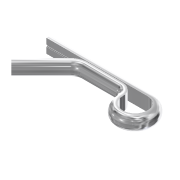
# Autodesk Inventor part: contra_pino_1
Saved by Autodesk Inventor 2012 SP2 (Build 160219200, 219)
## iProperties
Created: 2015-05-27
Part Number: contra_pino_1
Material: Default
Document SubType Name: Modeling
Designer: Projeto02
Density: 1 g/cm^3
Author: Projeto02
Autodesk Inventor part; units mm, degrees
ref_plane "YZ Plane" through (0, 0, 0) normal (1, 0, 0) x (0, 1, 0)
ref_plane "XZ Plane" through (0, 0, 0) normal (0, 1, 0) x (-1, 0, 0)
ref_plane "XY Plane" through (0, 0, 0) normal (0, 0, 1) x (1, 0, 0)
sketch "Esboço1" plane through (0, 0, 0) normal (0, 0, 1) x (1, 0, 0)
  line L0 (0, 0) -> (20.55, 0)
  line L1 (23, -2.45) -> (23, -2.55)
  line L2 (15.55, -0.1) -> (8.4497, -0.1)
  line L3 (5.9749, -1.1251) -> (0, -7.1)
  line L4 (18, -2.55) -> (18, -2.55)
  line L5 (20.45, -5) -> (20.55, -5)
  arc A0 (23, -2.45) -> (20.55, 0) centre (20.55, -2.45) ccw
  arc A1 (20.55, -5) -> (23, -2.55) centre (20.55, -2.55) ccw
  arc A2 (18, -2.55) -> (20.45, -5) centre (20.45, -2.55) ccw
  arc A3 (18, -2.55) -> (15.55, -0.1) centre (15.55, -2.55) ccw
  arc A4 (8.4497, -0.1) -> (5.9749, -1.1251) centre (8.4497, -3.6) ccw
  point P0 (23, 0)
  point P1 (18, -0.1)
  point P2 (7, -0.1)
  dimension "d0" = 23
  dimension "d1" = 135
  dimension "d2" = 5
  dimension "d3" = 5
  dimension "d4" = 11
  dimension "d5" = 0.1
  dimension "d6" = 2.45
  dimension "d10" = 3.5
  constraints: 12 end point, 10 point on circle, 10 tangent, 6 point on line, 5 centre point, 3 equal radius, 2 parallel, 1 horizontal, 1 vertical, 1 vertical alignment
  measures "d0" distance of L0.start point (23, 0)
  measures "d1" angle of L2 L3
  measures "d2" distance between parallel lines of L0 L5
  measures "d3" distance between parallel lines of L1 L4
  measures "d4" distance of point (18, -0.1) point (7, -0.1)
  measures "d5" distance between parallel lines of L0 L2
  measures "d6" radius of A0
  measures "d10" radius of A4
sketch "Esboço2" plane through (0, 0, 0) normal (1, 0, 0) x (0, 1, 0)
  line L0 (0, -1.5038) -> (0, 1.2962)
  line L1 (0, 1.2962) -> (0.15, 1.2962)
  line L2 (1.4, 0.0462) -> (1.4, -0.2538)
  line L3 (0.15, -1.5038) -> (0, -1.5038)
  arc A0 (1.4, 0.0462) -> (0.15, 1.2962) centre (0.15, 0.0462) ccw
  arc A1 (0.15, -1.5038) -> (1.4, -0.2538) centre (0.15, -0.2538) ccw
  dimension "d13" = 2.8
  dimension "d14" = 90
  dimension "d15" = 90
  dimension "d16" = 1.4
  dimension "d17" = 1.25
  constraints: 8 end point, 4 point on circle, 4 tangent, 2 centre point, 1 equal radius, 1 parallel
  measures "d13" distance of L0.start L0.end
  measures "d14" angle of L2 L3
  measures "d15" angle of L1 L2
  measures "d16" distance between parallel lines of L0 L2
  measures "d17" radius of A0
sweep "Varredura1" add profiles "Esboço2" path "Esboço1"
sketch "Esboço3" plane through (0, 0, -1.5038) normal (-1, 0, 0) x (0, 0, 1)
  line L0 (0, 0) -> (2.8, 0) projected
  circle A0 centre (1.4, -0.05) radius 0.2272
  point P0 (1.5038, 0)
  dimension "d18" = 1.4
  dimension "d19" = 2.8
  dimension "d20" = 0.05
  constraints: 1 centre point
  measures "d18" horizontal distance of L0.start A0.centre
  measures "d19" distance of L0.start L0.end
  measures "d20" distance from line of L0 A0.centre
extrude "Extrusão1" cut sketch "Esboço3" against normal blind 15.05
equation "\"d3\" = d2"
equation "\"d13\" = 2 * d16"
equation "\"d15\" = d14"
equation "\"d18\" = 0.5 * d19"
